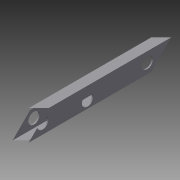
# Autodesk Inventor part: side 1
Saved by Autodesk Inventor 2015 (Build 190159000, 159)
## iProperties
Created: 2014-07-12
Part Number: side 1
Material: Generic
Document SubType Name: Modeling
Designer: admin
Density: 1 g/cm^3
Appearance: Default
Author: admin
Autodesk Inventor part; units mm, degrees
ref_plane "YZ Plane" through (0, 0, 0) normal (1, 0, 0) x (0, 1, 0)
ref_plane "XZ Plane" through (0, 0, 0) normal (0, 1, 0) x (-1, 0, 0)
ref_plane "XY Plane" through (0, 0, 0) normal (0, 0, 1) x (1, 0, 0)
sketch "Sketch1" plane through (0, 0, 0) normal (0, 0, 1) x (1, 0, 0)
  line L0 (9.525, 22.225) -> (9.525, -22.225)
  line L1 (9.525, -22.225) -> (-9.525, -22.225)
  line L2 (-9.525, -22.225) -> (-9.525, 22.225)
  line L3 (-9.525, 22.225) -> (9.525, 22.225)
  line L4 (12.7, 25.4) -> (-12.7, 25.4)
  line L5 (-12.7, 25.4) -> (-12.7, -25.4)
  line L6 (-12.7, -25.4) -> (12.7, -25.4)
  line L7 (12.7, -25.4) -> (12.7, 25.4)
  point P0 (0, 0)
  point P1 (0, 0)
  constraints: 16 end point
extrude "Extrusion1" add sketch "Sketch1" along normal blind 393.7
sketch "Sketch2" plane through (12.7, -25.4, 0) normal (1, 0, 0) x (0, 0, -1)
  circle A0 centre (-215.9, 18.9017) radius 14.2875
  point P0 (0, 25.4)
  dimension "d2" = 28.575
  constraints: 1 centre point
  measures "d2" diameter of A0
extrude "Extrusion2" cut sketch "Sketch2" against normal blind 25.4
sketch "Sketch3" plane through (12.7, -25.4, 0) normal (1, 0, 0) x (0, 0, -1)
  circle A0 centre (-215.9, 18.9017) radius 14.2875 projected
  circle A1 centre (-330.2, 25.4) radius 14.2875
  circle A2 centre (-63.5, 25.4) radius 14.2875
  line L0 (-393.7, 0) -> (-393.7, 50.8) projected
  line L1 (0, 0) -> (0, 50.8) projected
  point P0 (0, 25.4)
  dimension "d10" = 28.575
  dimension "d13" = 28.575
  dimension "d17" = 6.4983
  dimension "d20" = 63.5
  dimension "d21" = 63.5
  constraints: 2 centre point
  measures "d10" diameter of A1
  measures "d13" diameter of A2
  measures "d17" vertical distance of A1.centre A0.centre
  measures "d20" distance from line of L0 A1.centre
  measures "d21" distance from line of L1 A2.centre
extrude "Extrusion3" cut sketch "Sketch3" against normal blind 25.4 contours A1 | A2
body "Solid1"
